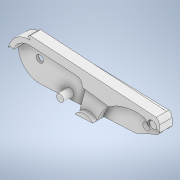
# Autodesk Inventor part: Pieza1
Saved by Autodesk Inventor 2022 (Build 260153000, 153)
## iProperties
Created: 2022-11-04
Part Number: Pieza1
Material: Resina acetálica, blanca
Document SubType Name: Modeling
Designer: Mauricio Guerrero
Density: 1.425 g/cm^3
Appearance: Suave - Blanco
Author: Mauricio Guerrero
Autodesk Inventor part; units mm, degrees
ref_plane "YZ Plane" through (0, 0, 0) normal (1, 0, 0) x (0, 1, 0)
ref_plane "XZ Plane" through (0, 0, 0) normal (0, 1, 0) x (-1, 0, 0)
ref_plane "XY Plane" through (0, 0, 0) normal (0, 0, 1) x (1, 0, 0)
sketch "Boceto1" plane through (0, 0, 0) normal (0, 0, 1) x (1, 0, 0)
  circle A0 centre (8.9388, 9.1447) radius 1.25
  circle A1 centre (47.9388, 9.1447) radius 1.25
  arc A2 (9.1664, 16.6413) -> (9.3419, 1.6556) centre (8.9388, 9.1447) ccw
  line L0 (8.9388, 9.1447) -> (47.9388, 9.1447) construction
  arc A3 (48.2289, 6.1588) -> (50.9361, 9.271) centre (47.9388, 9.1447) ccw
  circle A4 centre (51.4388, 12.1447) radius 1.25
  line L1 (53.9388, 11.1447) -> (53.9388, 13.5511)
  line L2 (51.4388, 12.1447) -> (51.4388, 15.3947) construction
  line L3 (51.4388, 12.1447) -> (51.4388, 10.1447) construction
  arc A5 (53.9388, 13.5511) -> (52.8836, 15.3138) centre (51.9388, 13.5511) ccw
  line L4 (9.1664, 16.6413) -> (52.8836, 15.3138)
  line L5 (42.8032, 3.438) -> (42.2388, 3.4264) construction
  line L6 (42.2388, 3.4264) -> (9.3419, 1.6556)
  line L7 (42.2388, 3.4264) -> (48.2289, 6.1588)
  arc A6 (51.4388, 10.1447) -> (50.9388, 9.1447) centre (52.0171, 9.2306) ccw
  line L8 (51.4388, 10.1447) -> (52.4166, 10.1447)
  arc A7 (52.4166, 10.1447) -> (53.9388, 11.1447) centre (52.4554, 11.7442) ccw
  point P0 (53.9388, 10.1447)
  point P1 (53.9388, 14.1447)
  dimension "d9" = 2.5
  dimension "d10" = 2.5
  dimension "d11" = 39
  dimension "d12" = 15
  dimension "d13" = 6
  dimension "d14" = 2.5
  dimension "d15" = 3.5
  dimension "d16" = 3
  dimension "d17" = 4
  dimension "d18" = 2.5
  dimension "d19" = 3.25
  dimension "d20" = 2
  dimension "d21" = 2
  dimension "d22" = 5.6
  dimension "d23" = 5.7
  constraints: 18 end point, 13 point on circle, 8 centre point, 3 tangent, 3 vertical, 2 coincident, 2 point on line, 1 horizontal, 1 horizontal alignment
  measures "d9" diameter of A0
  measures "d10" diameter of A1
  measures "d11" distance of L0.end A0.centre
  measures "d12" diameter of A2
  measures "d13" diameter of A3
  measures "d14" diameter of A4
  measures "d15" horizontal distance of L0.end L2.start
  measures "d16" vertical distance of L2.start L0.end
  measures "d17" distance of point (53.939, 10.145) point (53.939, 14.145)
  measures "d18" distance from line of L1 L2.start
  measures "d19" distance of L2.start L2.end
  measures "d20" distance of L3.end L2.start
  measures "d21" radius of A5
  measures "d22" distance from line of L0.end L5
  measures "d23" horizontal distance of L0.end L5.end
extrude "Extrusión1" add sketch "Boceto1" along normal blind 0.8 contours A1 | L4 A5 L1 A7 L8 A6 A3 L7 L6 A2
sketch "Boceto2" plane through (0, 0, 0.8) normal (0, 0, 1) x (1, 0, 0)
  circle A0 centre (8.9388, 9.1447) radius 1.25 projected
  arc A1 (9.5209, 14.9811) -> (3.3406, 10.8947) centre (8.9388, 9.1447) ccw
  arc A2 (9.1664, 16.6413) -> (1.5921, 10.6536) centre (8.9388, 9.1447) ccw
  circle A3 centre (51.4388, 12.1447) radius 1.25 projected
  arc A4 (52.9625, 11.7826) -> (50.031, 11.4584) centre (51.4388, 12.1447) ccw
  arc A5 (53.9388, 11.1447) -> (52.9625, 11.7826) centre (53.174, 11.0403) ccw
  arc A6 (53.9388, 13.5511) -> (52.8836, 15.3138) centre (51.9388, 13.5511) ccw projected
  line L0 (53.9388, 11.1447) -> (53.9388, 13.5511)
  arc A7 (53.9388, 13.5511) -> (52.4126, 15.3281) centre (52.1411, 13.5511) ccw
  line L1 (50.031, 11.4584) -> (48.9375, 13.1277)
  arc A8 (48.9375, 13.1277) -> (30.8534, 2.5471) centre (45.9501, -2.5111) ccw
  circle A9 centre (51.4388, 12.1447) radius 1.25
  circle A10 centre (19.4998, 4.4083) radius 1.25
  line L2 (30.8534, 2.5471) -> (24.6623, 2.2138)
  line L3 (24.6623, 2.2138) -> (27.1021, 11.5399)
  arc A11 (27.1021, 11.5399) -> (25.1673, 14.0461) centre (25.1673, 12.0461) ccw
  line L4 (9.1664, 16.6413) -> (8.4891, 17.498)
  line L5 (8.4891, 17.498) -> (9.1664, 18.0334)
  line L6 (9.1664, 18.0334) -> (52.8836, 15.3138)
  arc A12 (3.3406, 10.8947) -> (1.5921, 10.6536) centre (2.5355, 10.2725) ccw
  line L7 (25.1673, 14.0461) -> (9.5209, 14.9811)
  point P0 (0, 0)
  point P1 (1.4388, 9.1447)
  point P2 (23.6867, 2.4277)
  dimension "d35" = 2.5
  dimension "d36" = 2
  constraints: 17 point on circle, 16 end point, 10 centre point, 4 coincident, 3 tangent, 1 concentric, 1 perpendicular, 1 vertical
  measures "d35" diameter of A10
  measures "d36" radius of A11
extrude "Extrusión2" add sketch "Boceto2" along normal blind 2 contours A1 A12 A2 L4 L5 L6 A6 L0 A5 A4 L1 A8 L2 L3 A11 L7 | A10
sketch "Boceto3" plane through (0, 0, 0) normal (0, 0, -1) x (-1, 0, 0)
  circle A0 centre (-51.4388, 12.1447) radius 1.25 projected
  circle A1 centre (-51.4388, 12.1447) radius 1.25
  circle A2 centre (-19.4998, 4.4083) radius 1.25 projected
  circle A3 centre (-19.4998, 4.4083) radius 1.25
  circle A4 centre (-47.7976, 7.8947) radius 1.25
  point P0 (0, 0)
  dimension "d39" = 2.5
  constraints: 3 centre point, 2 coincident
  measures "d39" diameter of A4
extrude "Extrusión3" add sketch "Boceto3" against normal blind 4 contours A0 | A2
sketch "Boceto7" plane through (0, 0, 0.8) normal (0, 0, 1) x (1, 0, 0)
  circle A0 centre (46.86, 8.2808) radius 1.25
  point P0 (0, 0)
  dimension "d40" = 2.5
  constraints: 1 centre point
  measures "d40" diameter of A0
extrude "Extrusión6" add sketch "Boceto7" along normal blind 1
sketch "Boceto8" plane through (19.4998, 4.4083, 4) normal (0, 0, 1) x (1, 0, 0)
  circle A0 centre (0, 0) radius 1.25 projected
  circle A1 centre (0, 0) radius 1.25
  point P0 (-19.4998, -4.4083)
  constraints: 1 centre point, 1 coincident
extrude "Extrusión7" add sketch "Boceto8" along normal blind 0.4
sketch "Boceto9" plane through (0, 0, 2.8) normal (0, 0, 1) x (1, 0, 0)
  circle A0 centre (8.9388, 9.1447) radius 1.25
  arc A1 (9.5209, 14.9811) -> (3.3406, 10.8947) centre (8.9388, 9.1447) ccw
  arc A2 (9.1664, 16.6413) -> (1.5921, 10.6536) centre (8.9388, 9.1447) ccw
  circle A3 centre (51.4388, 12.1447) radius 1.25
  arc A4 (52.9625, 11.7826) -> (50.031, 11.4584) centre (51.4388, 12.1447) ccw
  arc A5 (53.9388, 11.1447) -> (52.9625, 11.7826) centre (53.174, 11.0403) ccw
  arc A6 (53.9388, 13.5511) -> (52.8836, 15.3138) centre (51.9388, 13.5511) ccw
  line L0 (53.9388, 11.1447) -> (53.9388, 13.5511)
  arc A7 (53.9388, 13.5511) -> (52.4126, 15.3281) centre (52.1411, 13.5511) ccw
  line L1 (50.031, 11.4584) -> (48.9375, 13.1277)
  arc A8 (48.9375, 13.1277) -> (36.4593, 10.2725) centre (45.9501, -2.5111) ccw
  circle A9 centre (51.4388, 12.1447) radius 1.25
  circle A10 centre (19.4998, 4.4083) radius 1.25
  arc A11 (27.1021, 11.5399) -> (25.1673, 14.0461) centre (25.1673, 12.0461) ccw
  line L2 (9.1664, 16.6413) -> (8.4891, 17.498)
  line L3 (8.4891, 17.498) -> (9.1664, 18.0334)
  line L4 (9.1664, 18.0334) -> (52.8836, 15.3138)
  arc A12 (3.3406, 10.8947) -> (1.5921, 10.6536) centre (2.5355, 10.2725) ccw
  line L5 (25.1673, 14.0461) -> (9.5209, 14.9811)
  line L6 (27.1021, 11.5399) -> (36.4593, 10.2725)
  line L7 (24.6623, 2.2138) -> (30.8534, 2.5471) projected
  line L8 (24.6623, 2.2138) -> (30.8534, 2.5471)
  arc A13 (30.9471, 2.8186) -> (30.8534, 2.5471) centre (45.9501, -2.5111) ccw projected
  arc A14 (30.8534, 2.5471) -> (24.6623, 2.2138) centre (27.8843, 0.03) ccw
  point P0 (0, 0)
  point P1 (1.4388, 9.1447)
  dimension "d45" = 2.5
  dimension "d46" = 2
  constraints: 21 point on circle, 16 end point, 14 centre point, 4 coincident, 2 tangent, 1 collinear, 1 concentric, 1 perpendicular, 1 vertical
  measures "d45" diameter of A10
  measures "d46" radius of A11
extrude "Extrusión8" add sketch "Boceto9" along normal blind 1.6 contours A1 A12 A2 L2 L3 L4 A6 L0 A5 A4 L1 A8 L6 A11 L5 | A14 L7
